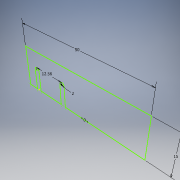
# Autodesk Inventor part: C2
Saved by Autodesk Inventor 2019 (Build 230136000, 136)
## iProperties
Created: 2020-03-27
Part Number: C2
Material: Generic
Document SubType Name: Modeling
Designer: Pulag
Density: 1 g/cm^3
Appearance: Default
Author: Pulag
Autodesk Inventor part; units mm, degrees
ref_plane "YZ Plane" through (0, 0, 0) normal (1, 0, 0) x (0, 1, 0)
ref_plane "XZ Plane" through (0, 0, 0) normal (0, 1, 0) x (-1, 0, 0)
ref_plane "XY Plane" through (0, 0, 0) normal (0, 0, 1) x (1, 0, 0)
sketch "Sketch1" plane through (0, 0, 0) normal (0, 0, 1) x (1, 0, 0)
  line L0 (45, 15) -> (-5, 15)
  line L1 (-1, 8) -> (-1, 0)
  line L2 (1, 0) -> (1, 8)
  arc A0 (1, 8) -> (-1, 8) centre (0, 8) ccw
  arc A1 (17, 8) -> (15, 8) centre (16, 8) ccw
  line L3 (15, 8) -> (15, 0)
  line L4 (17, 0) -> (17, 8)
  line L5 (2.5, 0) -> (2.5, 0)
  line L6 (22.48, 0) -> (22.48, 0)
  line L7 (-5, 15) -> (-5, 0)
  line L8 (-5, 0) -> (-1, 0)
  line L9 (45, 0) -> (45, 15)
  line L10 (17, 0) -> (45, 0)
  line L11 (1, 0) -> (15, 0)
  point P0 (0, 0)
  point P1 (15, 0)
  dimension "d0" = 50
  dimension "d1" = 15
  dimension "d3" = 2
  dimension "d6" = 0
  dimension "d7" = 16
  constraints: 24 end point, 6 point on line, 4 point on circle, 3 parallel, 2 centre point, 2 horizontal, 2 tangent, 2 vertical, 1 perpendicular
  measures "d0" distance of L0.end L0.start
  measures "d1" distance of L0.start L9.start
  measures "d3" diameter of A1
  measures "d6" distance of L6.start L6.end
  measures "d7" distance of A0.centre A1.centre
extrude "Extrusion2" add sketch "Sketch1" along normal blind 3.5
body "Solid2"
